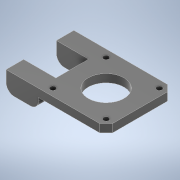
# Autodesk Inventor part: Zmotorsupport
Saved by Autodesk Inventor 2022 (Build 260153000, 153)
## iProperties
Created: 2022-02-20
Part Number: Zmotorsupport
Material: Genérico
Document SubType Name: Modeling
Designer: JK
Density: 1 g/cm^3
Appearance: Suave - Negro
Author: JK
Autodesk Inventor part; units mm, degrees
ref_plane "YZ Plane" through (0, 0, 0) normal (1, 0, 0) x (0, 1, 0)
ref_plane "XZ Plane" through (0, 0, 0) normal (0, 1, 0) x (-1, 0, 0)
ref_plane "XY Plane" through (0, 0, 0) normal (0, 0, 1) x (1, 0, 0)
sketch "Boceto1" plane through (0, 0, 0) normal (0, 1, 0) x (-1, 0, 0)
  line L0 (-21, 21) -> (21, 21)
  line L1 (21, 21) -> (21, -21)
  line L2 (21, -21) -> (-21, -21)
  line L3 (-21, -21) -> (-21, 21)
  line L4 (-21, 21) -> (21, -21) construction
  line L5 (21, 21) -> (-21, -21) construction
  circle A0 centre (0, 0) radius 11.1
  dimension "d0" = 42
  dimension "d1" = 42
  dimension "d2" = 22.2
  constraints: 12 end point, 2 midpoint, 2 parallel, 1 centre point, 1 coincident, 1 horizontal, 1 perpendicular
  measures "d0" distance of L0.end L1.end
  measures "d1" distance of L1.end L2.end
  measures "d2" diameter of A0
extrude "Extrusión1" add sketch "Boceto1" along normal blind 5
sketch "Boceto2" plane through (0, 5, 0) normal (0, 1, 0) x (1, 0, 0)
  line L0 (-21, 21) -> (-21, -21) projected
  line L1 (-21, -21) -> (-41, -21)
  line L2 (-41, -21) -> (-41, -10.15)
  line L3 (-41, -10.15) -> (-21, -10.15)
  line L4 (-21, -10.15) -> (-21, -21)
  line L5 (21, 21) -> (-21, 21) projected
  line L6 (-21, 21) -> (-41, 21)
  line L7 (-41, 21) -> (-41, 10.15)
  line L8 (-41, 10.15) -> (-21, 10.15)
  line L9 (-21, 10.15) -> (-21, 21)
  point P0 (0, 0)
  dimension "d5" = 20
  dimension "d6" = 20.3
  constraints: 16 end point, 4 parallel, 2 collinear, 2 horizontal, 2 perpendicular
  measures "d5" distance between parallel lines of L2 L0
  measures "d6" distance between parallel lines of L8 L3
extrude "Extrusión2" add sketch "Boceto2" against normal blind 12
sketch "Boceto3" plane through (0, 0, 0) normal (0, -1, 0) x (1, 0, 0)
  circle A0 centre (16.5, 16.5) radius 1.65
  point P0 (0, 0)
  dimension "d9" = 3.3
  dimension "d10" = 16.5
  dimension "d11" = 16.5
  constraints: 1 centre point
  measures "d9" diameter of A0
  measures "d10" horizontal distance of point (0, 0) A0.centre
  measures "d11" horizontal distance of A0.centre point (0, 0)
extrude "Extrusión3" cut sketch "Boceto3" against normal through all
chamfer "Chaflán1" distance 1.5 angle 45 1 edges at (14.85, 0, 16.5)
pattern_circular "Patrón circular1" count 4 over 360 about axis through (0, 0, 0) along (0, 1, 0) of "Extrusión3", "Chaflán1"
fillet "Empalme1" radius 5 4 edges at (-41, -7, -15.575) (-21, -7, -15.575) (-21, -7, 15.575) (-41, -7, 15.575)
chamfer "Chaflán3" distance 4 angle 45 2 edges at (21, 2.5, -21) (21, 2.5, 21)
